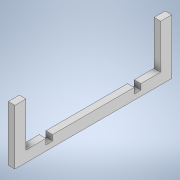
# Autodesk Inventor part: CONTAINERHOUDER LANG
Saved by Autodesk Inventor 2021 (Build 250183000, 183)
## iProperties
Created: 2022-02-02
Part Number: CONTAINERHOUDER LANG
Material: Generic
Document SubType Name: Modeling
Designer: ryan
Density: 1 g/cm^3
Appearance: Default
Author: ryan
Autodesk Inventor part; units mm, degrees
ref_plane "YZ Plane" through (0, 0, 0) normal (1, 0, 0) x (0, 1, 0)
ref_plane "XZ Plane" through (0, 0, 0) normal (0, 1, 0) x (-1, 0, 0)
ref_plane "XY Plane" through (0, 0, 0) normal (0, 0, 1) x (1, 0, 0)
sketch "Sketch1" plane through (0, 0, 0) normal (1, 0, 0) x (0, 1, 0)
  line L0 (0, 0) -> (0, -61)
  line L1 (0, -61) -> (20, -61)
  line L2 (20, -61) -> (20, -66)
  line L3 (20, -66) -> (-5, -66)
  line L4 (-5, -66) -> (-5, 5)
  line L5 (-5, 5) -> (20, 5)
  line L6 (20, 5) -> (20, 0)
  line L7 (20, 0) -> (0, 0)
  line L8 (0, -30.5) -> (0, -10.5)
  line L9 (0, -30.5) -> (0, -50.5)
  line L10 (0, -10.5) -> (0, -9)
  line L11 (0, -9) -> (-2.5, -9)
  line L12 (-2.5, -9) -> (-2.5, -12)
  line L13 (-2.5, -12) -> (0, -12)
  line L14 (0, -12) -> (0, -9)
  line L15 (0, -50.5) -> (0, -49)
  line L16 (0, -49) -> (-2.5, -49)
  line L17 (-2.5, -49) -> (-2.5, -52)
  line L18 (-2.5, -52) -> (0, -52)
  line L19 (0, -52) -> (0, -49)
  point P0 (0, -52)
  dimension "d0" = 61
  dimension "d1" = 20
  dimension "d2" = 5
  dimension "d3" = 25
  dimension "d4" = 71
  dimension "d7" = 20
  dimension "d8" = 20
  dimension "d9" = 1.5
  dimension "d10" = 2.5
  dimension "d11" = 3
  dimension "d12" = 1.5
  dimension "d13" = 2.5
  dimension "d14" = 3
  constraints: 40 end point, 6 perpendicular, 4 parallel, 4 point on line, 3 horizontal, 3 vertical, 1 midpoint
  measures "d0" distance of L0.start L0.end
  measures "d1" distance of L0.end L1.end
  measures "d2" distance of L1.end L2.end
  measures "d3" distance of L2.end L3.end
  measures "d4" distance of L3.end L4.end
  measures "d7" distance of L8.start L8.end
  measures "d8" distance of L8.start L9.end
  measures "d9" distance of L8.end L10.end
  measures "d10" distance of L13.end L12.end
  measures "d11" distance of L12.end L11.end
  measures "d12" distance of L9.end L15.end
  measures "d13" distance of L18.end L17.end
  measures "d14" distance of L17.end L16.end
extrude "Extrusion1" add sketch "Sketch1" along normal blind 3 contours L0 L11 L12 L13 L16 L17 L18 L1 L2 L3 L4 L5 L6 L7
body "Solid1"
